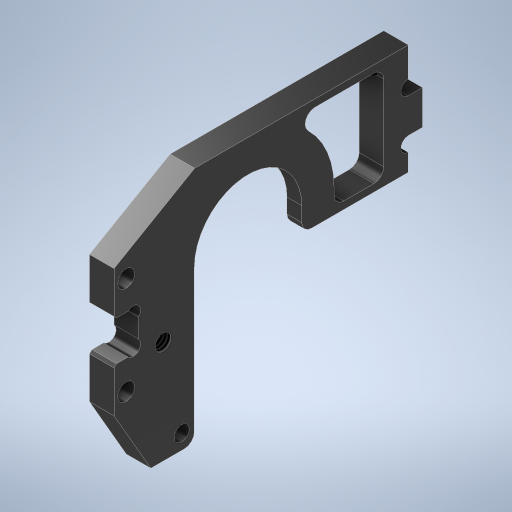
# Autodesk Inventor part: LegBaseSideFrame
Saved by Autodesk Inventor 2024.2 (Build 282272000, 272)
## iProperties
Created: 2024-01-07
Part Number: LegBaseSideFrame
Material: Aluminum 7075
Document SubType Name: Modeling
Designer: Masato Kubotera
Density: 2.81 g/cm^3
Appearance: Glossy - Black
Mass: 13.2467 g
Surface Area: 39.3099 cm^2
Volume: 4.71414 cm^3
Vendor: meviy
Author: Masato Kubotera
Autodesk Inventor part; units mm, degrees
ref_plane "YZ Plane" through (0, 0, 0) normal (1, 0, 0) x (0, 1, 0)
ref_plane "XZ Plane" through (0, 0, 0) normal (0, 1, 0) x (-1, 0, 0)
ref_plane "XY Plane" through (0, 0, 0) normal (0, 0, 1) x (1, 0, 0)
derived "LegBaseSideFrameBasis.ipt"
sketch "Sketch1" plane through (0, 0, 0) normal (0, 1, 0) x (-1, 0, 0)
  line L0 (0, 0) -> (17.3205, 10) construction
  line L1 (0, 0) -> (17.3205, 0) construction
  line L2 (17.3205, 22) -> (17.3205, -21) construction
  line L3 (33.3205, -21) -> (1.3205, -21) construction
  line L4 (1.3205, -21) -> (1.3205, 22) construction
  line L5 (1.3205, 22) -> (33.3205, 22) construction
  line L6 (33.3205, 22) -> (33.3205, -21) construction
  line L7 (33.3205, -21) -> (1.3205, 22) construction
  line L8 (1.3205, -21) -> (33.3205, 22) construction
  line L9 (30.8205, 9) -> (3.8205, 9) construction
  line L10 (3.8205, 9) -> (3.8205, -18) construction
  line L11 (3.8205, -18) -> (30.8205, -18) construction
  line L12 (30.8205, -18) -> (30.8205, 9) construction
  line L13 (30.8205, 9) -> (3.8205, -18) construction
  line L14 (3.8205, 9) -> (30.8205, -18) construction
  circle A0 centre (17.3205, 10) radius 8 construction
  line L15 (2.9205, -21) -> (2.9205, -32.5) construction
  line L16 (2.9205, -32.5) -> (31.7205, -32.5) construction
  line L17 (31.7205, -32.5) -> (31.7205, -21) construction
  line L18 (92.5, 16) -> (53, 16) construction
  line L19 (53, 16) -> (53, -27) construction
  line L20 (53, -27) -> (92.5, -27) construction
  line L21 (92.5, -27) -> (92.5, 16) construction
  line L22 (92.5, 16) -> (53, -27) construction
  line L23 (53, 16) -> (92.5, -27) construction
  line L24 (53, -23) -> (52.5, -23) construction
  line L25 (52.5, -23) -> (52.5, -7) construction
  line L26 (52.5, -7) -> (53, -7) construction
  line L27 (52.5, -15) -> (92.5, -15) construction
  line L28 (53, 0) -> (92.5, 0) construction
  line L29 (92.5, 16) -> (92.5, 27.5) construction
  line L30 (92.5, 27.5) -> (78.5, 27.5) construction
  line L31 (78.5, 27.5) -> (78.5, 16) construction
  arc A1 (28.2705, 10) -> (6.3705, 10) centre (17.3205, 10) ccw
  line L32 (6.3705, 10) -> (6.3705, -21)
  circle A2 centre (0, 0) radius 6 construction
  circle A3 centre (0, 0) radius 2 construction
  arc A4 (6.7375, 22) -> (1.3205, 10) centre (17.3205, 10) ccw construction
  arc A5 (5.8553, 21.2317) -> (1.2705, 10) centre (17.3205, 10) ccw
  line L33 (1.2705, 10) -> (1.2705, -21)
  arc A6 (7.7762, 22) -> (5.8553, 21.2317) centre (7.2191, 20.6073) ccw
  line L34 (-2.4944, -21) -> (-10, -8)
  line L35 (-10, -8) -> (-10, 0.95)
  line L36 (-10, 0.95) -> (-5, 0.95)
  line L37 (-5, 0.95) -> (-5, 9.05)
  line L38 (-5, 9.05) -> (-10, 9.05)
  line L39 (-10, 27.5) -> (52.9, 27.5)
  line L40 (-5, 5) -> (-10, 5) construction
  line L41 (92.5, 13) -> (53, 13) construction
  line L42 (92.5, -14) -> (53, -14) construction
  line L43 (21.45, 27.5) -> (21.45, -24.5252) construction
  line L44 (-5, 9) -> (-10, 9) construction
  line L45 (-5, 1) -> (-10, 1) construction
  arc A7 (28.7858, 21.2317) -> (26.8648, 22) centre (27.4219, 20.6073) ccw
  arc A8 (33.3705, 10) -> (28.7858, 21.2317) centre (17.3205, 10) ccw
  line L46 (33.3705, 10) -> (33.3705, 5)
  line L47 (52.9, 5) -> (28.2705, 5)
  line L48 (-2.4944, -21) -> (6.3705, -21)
  line L49 (28.2705, 10) -> (28.2705, 5)
  line L50 (-7.5, -5) -> (-7.5, 5) construction
  line L51 (-10, 27.5) -> (-10, 9)
  line L52 (6.6621, 22) -> (6.7375, 22)
  line L53 (7.7762, 22) -> (26.8648, 22)
  arc A9 (-5, 6.9287) -> (-7.1213, 9.05) centre (-6.0607, 7.9893) ccw
  arc A10 (-7.1213, 0.95) -> (-5, 3.0713) centre (-6.0607, 2.0107) ccw
  circle A11 centre (3.8205, -18) radius 1.55 construction
  line L54 (52.9, 5) -> (52.9, 27.5)
  line L55 (50, 27.5) -> (50, 18.5)
  line L56 (50, 18.5) -> (52.9, 18.5)
  line L57 (52.9, 11.5) -> (50, 11.5)
  line L58 (50, 11.5) -> (50, 5)
  arc A12 (50, 21.5) -> (50, 18.5) centre (50, 20) ccw
  arc A13 (50, 11.5) -> (50, 8.5) centre (50, 10) ccw
  line L59 (50, 24.5) -> (45, 24.5) construction
  line L60 (50, 21.5) -> (50, 27.5)
  line L61 (50, 8.5) -> (50, 5)
  line L62 (52.9, 18.5) -> (52.9, 11.5)
  line L63 (24.5318, 26) -> (45, 26)
  line L64 (45, 26) -> (45, 6.5)
  line L65 (45, 6.5) -> (34.8705, 6.5)
  line L66 (34.8705, 6.5) -> (34.8705, 10)
  arc A14 (34.8705, 10) -> (24.5318, 26) centre (17.3205, 10) ccw
  point P0 (17.3205, 0.5)
  point P1 (17.3205, -4.5)
  point P2 (17.3205, 0.5)
  point P3 (72.75, -5.5)
  point P4 (-7.5, 15)
  point P5 (27.979, 22)
  point P6 (8.8205, -21)
  point P7 (33.3705, 5.05)
  point P8 (1.2705, -21)
  point P9 (27.979, 22)
  point P10 (-5, 3.0713)
  point P11 (-7.1213, 0.95)
extrude "Extrusion1" add sketch "Sketch1" along normal blind 5 contours A1 L32 L48 L33 A5 A6 L53 A7 A8 L46 L47 L49 | L46 A8 A7 L53 A6 A5 L33 L48 L34 L35 L36 A10 L37 A9 L38 L51 L39 L55 A12 L56 L54 L57 A13 L58 L47
extrude "Extrusion3" cut sketch "Sketch1" along normal blind 2 contours A1 L32 L48 L33 A5 A6 L53 A7 A8 L46 L47 L49
hole "Phi3.5" at (7.5, 0, -5) at (7.5, 0, 15) direction (0, 1, 0) diameter 3.5 end through all
hole "Phi3.1" at (-30.8205, 0, -18) at (-3.8205, 0, -18) direction (0, 1, 0) diameter 3.1 end through all
hole "M4" at (0, 0, 0) direction (0, 1, 0) diameter 3.242 end through all counterbore diameter 4 counterbore depth 2 thread size "M4x0.7" class "6H" standard "ANSI Metric M Profile"
sketch "Sketch2" plane through (-50, 0, 21.5) normal (-1, 0, 0) x (0, 0, 1)
  line L0 (3, 0) -> (3, 5)
  line L1 (0, 5) -> (6, 5) projected
  point P0 (-21.5, 0)
  point P1 (3, 0)
  point P2 (3, 2.5)
  constraints: 2 end point, 2 midpoint, 1 vertical
hole "Side-M3" at (-50, 2.5, 24.5) direction (1, 0, 0) diameter 2.459 depth 6 thread size "M3x0.5" class "6H" standard "ANSI Metric M Profile"
chamfer "C0.5" distance 0.5 angle 45 2 edges at (10, 2.5, 9.05) (10, 2.5, 0.95)
fillet "R2" radius 2 8 edges at (-1.2705, 1, 1.5446) (-1.2705, 1, -1.5446) (-28.2705, 3.5, 5) (-6.3705, 3.5, -21) (-24.5318, 2.5, 26) (-45, 2.5, 26) (-34.8705, 2.5, 6.5) (-45, 2.5, 6.5)
chamfer "Chamfer1" distance 9.5 angle 60 1 edges at (10, 2.5, 27.5) measured on face at (10, 2.5, 27)
body "Solid1"
